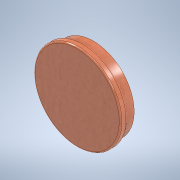
# Autodesk Inventor part: Mocowanie spadochronu
Saved by Autodesk Inventor 2020 (Build 240168000, 168)
## iProperties
Created: 2021-10-14
Part Number: Mocowanie spadochronu
Material: Ogólny
Document SubType Name: Modeling
Designer: Komputer
Density: 1 g/cm^3
Appearance: Orzech — naturalny — polerowany
Author: Komputer
Autodesk Inventor part; units mm, degrees
ref_plane "YZ Plane" through (0, 0, 0) normal (1, 0, 0) x (0, 1, 0)
ref_plane "XZ Plane" through (0, 0, 0) normal (0, 1, 0) x (-1, 0, 0)
ref_plane "XY Plane" through (0, 0, 0) normal (0, 0, 1) x (1, 0, 0)
sketch "Szkic1" plane through (0, 0, 0) normal (0, 0, 1) x (1, 0, 0)
  circle A0 centre (0, 0) radius 32
  dimension "d0" = 64
  constraints: 1 centre point, 1 coincident
  measures "d0" diameter of A0
extrude "Wyciągnięcie proste1" add sketch "Szkic1" along normal blind 5
sketch "Szkic2" plane through (0, 0, 0) normal (0, 0, -1) x (-1, 0, 0)
  circle A0 centre (0, 0) radius 5
  dimension "d3" = 10
  constraints: 1 centre point, 1 coincident
  measures "d3" diameter of A0
extrude "Wyciągnięcie proste2" add sketch "Szkic2" along normal blind 14
fillet "Zaokrąglenie1" radius 1 3 edges at (-32, 0, 0) (-32, 0, 5) (5, 0, -14)
sketch "Szkic3" plane through (0, 0, 0) normal (0, 0, -1) x (-1, 0, 0)
  circle A0 centre (0, 0) radius 27.5
  circle A1 centre (0, 0) radius 4 projected
  circle A2 centre (0, 0) radius 30
  line L0 (0, 26) -> (0.5, 26)
  line L1 (0, 26) -> (-0.5, 26)
  line L2 (-0.5, 26) -> (-1.3243, 27.4277)
  line L3 (-1.3243, 27.4277) -> (-1.347, 27.467)
  line L4 (0.5, 26) -> (1.347, 27.467)
  line L5 (-3.6185, 25.747) -> (-3.1234, 25.8166)
  line L6 (-3.6185, 25.747) -> (-4.1136, 25.6774)
  line L7 (-4.1136, 25.6774) -> (-5.1286, 26.9765)
  line L8 (-5.1286, 26.9765) -> (-5.1565, 27.0122)
  line L9 (-3.1234, 25.8166) -> (-2.4888, 27.3871)
  line L10 (-7.1666, 24.9928) -> (-6.6859, 25.1306)
  line L11 (-7.1666, 24.9928) -> (-7.6472, 24.855)
  line L12 (-7.6472, 24.855) -> (-8.8331, 26.0002)
  line L13 (-8.8331, 26.0002) -> (-8.8657, 26.0317)
  line L14 (-6.6859, 25.1306) -> (-6.2761, 26.7742)
  line L15 (-10.5752, 23.7522) -> (-10.1184, 23.9556)
  line L16 (-10.5752, 23.7522) -> (-11.0319, 23.5488)
  line L17 (-11.0319, 23.5488) -> (-12.3657, 24.5178)
  line L18 (-12.3657, 24.5178) -> (-12.4023, 24.5445)
  line L19 (-10.1184, 23.9556) -> (-9.9413, 25.6402)
  line L20 (-13.7779, 22.0493) -> (-13.3539, 22.3142)
  line L21 (-13.7779, 22.0493) -> (-14.2019, 21.7843)
  line L22 (-14.2019, 21.7843) -> (-15.6576, 22.5583)
  line L23 (-15.6576, 22.5583) -> (-15.6976, 22.5795)
  line L24 (-13.3539, 22.3142) -> (-13.413, 24.0071)
  line L25 (-16.7125, 19.9172) -> (-16.3295, 20.2385)
  line L26 (-16.7125, 19.9172) -> (-17.0955, 19.5958)
  line L27 (-17.0955, 19.5958) -> (-18.6447, 20.1596)
  line L28 (-18.6447, 20.1596) -> (-18.6873, 20.1751)
  line L29 (-16.3295, 20.2385) -> (-16.6236, 21.9068)
  line L30 (-19.3218, 17.3974) -> (-18.9872, 17.769)
  line L31 (-19.3218, 17.3974) -> (-19.6563, 17.0258)
  line L32 (-19.6563, 17.0258) -> (-21.2689, 17.3686)
  line L33 (-21.2689, 17.3686) -> (-21.3133, 17.378)
  line L34 (-18.9872, 17.769) -> (-19.5107, 19.38)
  line L35 (-21.555, 14.539) -> (-21.2754, 14.9535)
  line L36 (-21.555, 14.539) -> (-21.8346, 14.1245)
  line L37 (-21.8346, 14.1245) -> (-23.4792, 14.2395)
  line L38 (-23.4792, 14.2395) -> (-23.5244, 14.2427)
  line L39 (-21.2754, 14.9535) -> (-22.018, 16.476)
  line L40 (-23.3686, 11.3976) -> (-23.1495, 11.847)
  line L41 (-23.3686, 11.3976) -> (-23.5878, 10.9483)
  line L42 (-23.5878, 10.9483) -> (-25.2324, 10.8333)
  line L43 (-25.2324, 10.8333) -> (-25.2776, 10.8301)
  line L44 (-23.1495, 11.847) -> (-24.0967, 13.2514)
  line L45 (-24.7275, 8.0344) -> (-24.573, 8.51)
  line L46 (-24.7275, 8.0344) -> (-24.882, 7.5589)
  line L47 (-24.882, 7.5589) -> (-26.4946, 7.2161)
  line L48 (-26.4946, 7.2161) -> (-26.5389, 7.2067)
  line L49 (-24.573, 8.51) -> (-25.7064, 9.7688)
  line L50 (-25.605, 4.5149) -> (-25.5182, 5.0073)
  line L51 (-25.605, 4.5149) -> (-25.6918, 4.0224)
  line L52 (-25.6918, 4.0224) -> (-27.241, 3.4586)
  line L53 (-27.241, 3.4586) -> (-27.2836, 3.4431)
  line L54 (-25.5182, 5.0073) -> (-26.8158, 6.0961)
  line L55 (-25.9842, 0.9074) -> (-25.9667, 1.4071)
  line L56 (-25.9842, 0.9074) -> (-26.0016, 0.4077)
  line L57 (-26.0016, 0.4077) -> (-27.4573, -0.3663)
  line L58 (-27.4573, -0.3663) -> (-27.4973, -0.3876)
  line L59 (-25.9667, 1.4071) -> (-27.4033, 2.3047)
  line L60 (-25.8576, -2.7177) -> (-25.9098, -2.2205)
  line L61 (-25.8576, -2.7177) -> (-25.8053, -3.215)
  line L62 (-25.8053, -3.215) -> (-27.1391, -4.184)
  line L63 (-27.1391, -4.184) -> (-27.1757, -4.2107)
  line L64 (-25.9098, -2.2205) -> (-27.4573, -1.5315)
  line L65 (-25.2277, -6.29) -> (-25.3486, -5.8048)
  line L66 (-25.2277, -6.29) -> (-25.1067, -6.7751)
  line L67 (-25.1067, -6.7751) -> (-26.2926, -7.9203)
  line L68 (-26.2926, -7.9203) -> (-26.3252, -7.9518)
  line L69 (-25.3486, -5.8048) -> (-26.977, -5.3379)
  line L70 (-24.1068, -9.7398) -> (-24.2941, -9.2762)
  line L71 (-24.1068, -9.7398) -> (-23.9195, -10.2034)
  line L72 (-23.9195, -10.2034) -> (-24.9345, -11.5025)
  line L73 (-24.9345, -11.5025) -> (-24.9624, -11.5382)
  line L74 (-24.2941, -9.2762) -> (-25.9715, -9.0404)
  line L75 (-22.5167, -13) -> (-22.7667, -12.567)
  line L76 (-22.5167, -13) -> (-22.2667, -13.433)
  line L77 (-22.2667, -13.433) -> (-23.091, -14.8608)
  line L78 (-23.091, -14.8608) -> (-23.1136, -14.9)
  line L79 (-22.7667, -12.567) -> (-24.4606, -12.567)
  line L80 (-20.4883, -16.0072) -> (-20.7961, -15.6132)
  line L81 (-20.4883, -16.0072) -> (-20.1804, -16.4012)
  line L82 (-20.1804, -16.4012) -> (-20.798, -17.9298)
  line L83 (-20.798, -17.9298) -> (-20.815, -17.9718)
  line L84 (-20.7961, -15.6132) -> (-22.4736, -15.8489)
  line L85 (-18.0611, -18.7028) -> (-18.4208, -18.3555)
  line L86 (-18.0611, -18.7028) -> (-17.7014, -19.0502)
  line L87 (-17.7014, -19.0502) -> (-18.1003, -20.6498)
  line L88 (-18.1003, -20.6498) -> (-18.1112, -20.6938)
  line L89 (-18.4208, -18.3555) -> (-20.0491, -18.8224)
  line L90 (-15.2824, -21.0344) -> (-15.6869, -20.7405)
  line L91 (-15.2824, -21.0344) -> (-14.8779, -21.3283)
  line L92 (-14.8779, -21.3283) -> (-15.0502, -22.9679)
  line L93 (-15.0502, -22.9679) -> (-15.055, -23.013)
  line L94 (-15.6869, -20.7405) -> (-17.2344, -21.4295)
  line L95 (-12.2063, -22.9566) -> (-12.6477, -22.7219)
  line L96 (-12.2063, -22.9566) -> (-11.7648, -23.1914)
  line L97 (-11.7648, -23.1914) -> (-11.7073, -24.839)
  line L98 (-11.7073, -24.839) -> (-11.7057, -24.8843)
  line L99 (-12.6477, -22.7219) -> (-14.0843, -23.6196)
  line L100 (-8.8925, -24.432) -> (-9.3624, -24.261)
  line L101 (-8.8925, -24.432) -> (-8.4227, -24.603)
  line L102 (-8.4227, -24.603) -> (-8.1364, -26.2266)
  line L103 (-8.1364, -26.2266) -> (-8.1285, -26.2712)
  line L104 (-9.3624, -24.261) -> (-10.66, -25.3498)
  line L105 (-5.4057, -25.4318) -> (-5.8948, -25.3279)
  line L106 (-5.4057, -25.4318) -> (-4.9166, -25.5358)
  line L107 (-4.9166, -25.5358) -> (-4.4072, -27.1037)
  line L108 (-4.4072, -27.1037) -> (-4.3932, -27.1468)
  line L109 (-5.8948, -25.3279) -> (-7.0282, -26.5867)
  line L110 (-1.8137, -25.9367) -> (-2.3125, -25.9018)
  line L111 (-1.8137, -25.9367) -> (-1.3149, -25.9715)
  line L112 (-1.3149, -25.9715) -> (-0.5922, -27.4533)
  line L113 (-0.5922, -27.4533) -> (-0.5723, -27.494)
  line L114 (-2.3125, -25.9018) -> (-3.2597, -27.3061)
  line L115 (1.8137, -25.9367) -> (1.3149, -25.9715)
  line L116 (1.8137, -25.9367) -> (2.3125, -25.9018)
  line L117 (2.3125, -25.9018) -> (3.2343, -27.2686)
  line L118 (3.2343, -27.2686) -> (3.2597, -27.3061)
  line L119 (1.3149, -25.9715) -> (0.5723, -27.494)
  line L120 (5.4057, -25.4318) -> (4.9166, -25.5358)
  line L121 (5.4057, -25.4318) -> (5.8948, -25.3279)
  line L122 (5.8948, -25.3279) -> (6.9979, -26.553)
  line L123 (6.9979, -26.553) -> (7.0282, -26.5867)
  line L124 (4.9166, -25.5358) -> (4.3932, -27.1468)
  line L125 (8.8925, -24.432) -> (8.4227, -24.603)
  line L126 (8.8925, -24.432) -> (9.3624, -24.261)
  line L127 (9.3624, -24.261) -> (10.6253, -25.3207)
  line L128 (10.6253, -25.3207) -> (10.66, -25.3498)
  line L129 (8.4227, -24.603) -> (8.1285, -26.2712)
  line L130 (12.2063, -22.9566) -> (11.7648, -23.1914)
  line L131 (12.2063, -22.9566) -> (12.6477, -22.7219)
  line L132 (12.6477, -22.7219) -> (14.0458, -23.5955)
  line L133 (14.0458, -23.5955) -> (14.0843, -23.6196)
  line L134 (11.7648, -23.1914) -> (11.7057, -24.8843)
  line L135 (15.2824, -21.0344) -> (14.8779, -21.3283)
  line L136 (15.2824, -21.0344) -> (15.6869, -20.7405)
  line L137 (15.6869, -20.7405) -> (17.193, -21.4111)
  line L138 (17.193, -21.4111) -> (17.2344, -21.4295)
  line L139 (14.8779, -21.3283) -> (15.055, -23.013)
  line L140 (18.0611, -18.7028) -> (17.7014, -19.0502)
  line L141 (18.0611, -18.7028) -> (18.4208, -18.3555)
  line L142 (18.4208, -18.3555) -> (20.0055, -18.8099)
  line L143 (20.0055, -18.8099) -> (20.0491, -18.8224)
  line L144 (17.7014, -19.0502) -> (18.1112, -20.6938)
  line L145 (20.4883, -16.0072) -> (20.1804, -16.4012)
  line L146 (20.4883, -16.0072) -> (20.7961, -15.6132)
  line L147 (20.7961, -15.6132) -> (22.4287, -15.8426)
  line L148 (22.4287, -15.8426) -> (22.4736, -15.8489)
  line L149 (20.1804, -16.4012) -> (20.815, -17.9718)
  line L150 (22.5167, -13) -> (22.2667, -13.433)
  line L151 (22.5167, -13) -> (22.7667, -12.567)
  line L152 (22.7667, -12.567) -> (24.4153, -12.567)
  line L153 (24.4153, -12.567) -> (24.4606, -12.567)
  line L154 (22.2667, -13.433) -> (23.1136, -14.9)
  line L155 (24.1068, -9.7398) -> (23.9195, -10.2034)
  line L156 (24.1068, -9.7398) -> (24.2941, -9.2762)
  line L157 (24.2941, -9.2762) -> (25.9267, -9.0467)
  line L158 (25.9267, -9.0467) -> (25.9715, -9.0404)
  line L159 (23.9195, -10.2034) -> (24.9624, -11.5382)
  line L160 (25.2277, -6.29) -> (25.1067, -6.7751)
  line L161 (25.2277, -6.29) -> (25.3486, -5.8048)
  line L162 (25.3486, -5.8048) -> (26.9334, -5.3504)
  line L163 (26.9334, -5.3504) -> (26.977, -5.3379)
  line L164 (25.1067, -6.7751) -> (26.3252, -7.9518)
  line L165 (25.8576, -2.7177) -> (25.8053, -3.215)
  line L166 (25.8576, -2.7177) -> (25.9098, -2.2205)
  line L167 (25.9098, -2.2205) -> (27.4159, -1.5499)
  line L168 (27.4159, -1.5499) -> (27.4573, -1.5315)
  line L169 (25.8053, -3.215) -> (27.1757, -4.2107)
  line L170 (25.9842, 0.9074) -> (26.0016, 0.4077)
  line L171 (25.9842, 0.9074) -> (25.9667, 1.4071)
  line L172 (25.9667, 1.4071) -> (27.3648, 2.2807)
  line L173 (27.3648, 2.2807) -> (27.4033, 2.3047)
  line L174 (26.0016, 0.4077) -> (27.4973, -0.3876)
  line L175 (25.605, 4.5149) -> (25.6918, 4.0224)
  line L176 (25.605, 4.5149) -> (25.5182, 5.0073)
  line L177 (25.5182, 5.0073) -> (26.7811, 6.067)
  line L178 (26.7811, 6.067) -> (26.8158, 6.0961)
  line L179 (25.6918, 4.0224) -> (27.2836, 3.4431)
  line L180 (24.7275, 8.0344) -> (24.882, 7.5589)
  line L181 (24.7275, 8.0344) -> (24.573, 8.51)
  line L182 (24.573, 8.51) -> (25.6761, 9.7351)
  line L183 (25.6761, 9.7351) -> (25.7064, 9.7688)
  line L184 (24.882, 7.5589) -> (26.5389, 7.2067)
  line L185 (23.3686, 11.3976) -> (23.5878, 10.9483)
  line L186 (23.3686, 11.3976) -> (23.1495, 11.847)
  line L187 (23.1495, 11.847) -> (24.0714, 13.2138)
  line L188 (24.0714, 13.2138) -> (24.0967, 13.2514)
  line L189 (23.5878, 10.9483) -> (25.2776, 10.8301)
  line L190 (21.555, 14.539) -> (21.8346, 14.1245)
  line L191 (21.555, 14.539) -> (21.2754, 14.9535)
  line L192 (21.2754, 14.9535) -> (21.9981, 16.4353)
  line L193 (21.9981, 16.4353) -> (22.018, 16.476)
  line L194 (21.8346, 14.1245) -> (23.5244, 14.2427)
  line L195 (19.3218, 17.3974) -> (19.6563, 17.0258)
  line L196 (19.3218, 17.3974) -> (18.9872, 17.769)
  line L197 (18.9872, 17.769) -> (19.4967, 19.3369)
  line L198 (19.4967, 19.3369) -> (19.5107, 19.38)
  line L199 (19.6563, 17.0258) -> (21.3133, 17.378)
  line L200 (16.7125, 19.9172) -> (17.0955, 19.5958)
  line L201 (16.7125, 19.9172) -> (16.3295, 20.2385)
  line L202 (16.3295, 20.2385) -> (16.6157, 21.8621)
  line L203 (16.6157, 21.8621) -> (16.6236, 21.9068)
  line L204 (17.0955, 19.5958) -> (18.6873, 20.1751)
  line L205 (13.7779, 22.0493) -> (14.2019, 21.7843)
  line L206 (13.7779, 22.0493) -> (13.3539, 22.3142)
  line L207 (13.3539, 22.3142) -> (13.4114, 23.9618)
  line L208 (13.4114, 23.9618) -> (13.413, 24.0071)
  line L209 (14.2019, 21.7843) -> (15.6976, 22.5795)
  line L210 (10.5752, 23.7522) -> (11.0319, 23.5488)
  line L211 (10.5752, 23.7522) -> (10.1184, 23.9556)
  line L212 (10.1184, 23.9556) -> (9.9461, 25.5951)
  line L213 (9.9461, 25.5951) -> (9.9413, 25.6402)
  line L214 (11.0319, 23.5488) -> (12.4023, 24.5445)
  line L215 (7.1666, 24.9928) -> (7.6472, 24.855)
  line L216 (7.1666, 24.9928) -> (6.6859, 25.1306)
  line L217 (6.6859, 25.1306) -> (6.2871, 26.7303)
  line L218 (6.2871, 26.7303) -> (6.2761, 26.7742)
  line L219 (7.6472, 24.855) -> (8.8657, 26.0317)
  line L220 (3.6185, 25.747) -> (4.1136, 25.6774)
  line L221 (3.6185, 25.747) -> (3.1234, 25.8166)
  line L222 (3.1234, 25.8166) -> (2.5058, 27.3451)
  line L223 (2.5058, 27.3451) -> (2.4888, 27.3871)
  line L224 (4.1136, 25.6774) -> (5.1565, 27.0122)
  point P0 (27.4973, -0.3876)
  dimension "d7" = 55
  dimension "d8" = 60
  dimension "d16" = 0.5
  dimension "d17" = 0.5
  dimension "d18" = 120
  dimension "d22" = 360
  constraints: 450 end point, 45 point on line, 2 coincident, 1 centre point, 1 horizontal, 499 other
  measures "d8" diameter of A2
  measures "d16" distance of L0.start L0.end
  measures "d17" distance of L0.start L1.end
  measures "d18" angle of L1 L2
extrude "Wyciągnięcie proste3" add sketch "Szkic3" along normal blind 7 contours A0 L174 L170 L171 L172 L173 | L179 L175 L176 L177 L178 A0 | A0 L169 L165 L166 L167 L168 | L184 L180 L181 L182 L183 A0 | A0 L164 L160 L161 L162 L163 | L189 L185 L186 L187 L188 A0 | A0 L159 L155 L156 L157 L158 | L194 L190 L191 L192 L193 A0 | A0 L154 L150 L151 L152 L153 | L199 L195 L196 L197 L198 A0 | A0 L149 L145 L146 L147 L148 | L204 L200 L201 L202 L203 A0 | A0 L144 L140 L141 L142 L143 | L209 L205 L206 L207 L208 A0 | A0 L139 L135 L136 L137 L138 | L214 L210 L211 L212 L213 A0 | A0 L134 L130 L131 L132 L133 | L219 L215 L216 L217 L218 A0 | A0 L129 L125 L126 L127 L128 | L224 L220 L221 L222 L223 A0 | A0 L124 L120 L121 L122 L123 | L4 L0 L1 L2 L3 A0 | A0 L119 L115 L116 L117 L118 | L9 L5 L6 L7 L8 A0 | A0 L114 L110 L111 L112 L113 | L14 L10 L11 L12 L13 A0 | A0 L109 L105 L106 L107 L108 | L19 L15 L16 L17 L18 A0 | A0 L104 L100 L101 L102 L103 | L24 L20 L21 L22 L23 A0 | A0 L99 L95 L96 L97 L98 | L29 L25 L26 L27 L28 A0 | A0 L94 L90 L91 L92 L93 | L34 L30 L31 L32 L33 A0 | A0 L89 L85 L86 L87 L88 | L39 L35 L36 L37 L38 A0 | A0 L84 L80 L81 L82 L83 | L44 L40 L41 L42 L43 A0 | A0 L79 L75 L76 L77 L78 | L49 L45 L46 L47 L48 A0 | A0 L74 L70 L71 L72 L73 | L54 L50 L51 L52 L53 A0 | A0 L69 L65 L66 L67 L68 | L59 L55 L56 L57 L58 A0 | A0 L64 L60 L61 L62 L63 | A2
sketch "Szkic4" plane through (0, 0, -14) normal (0, 0, -1) x (-1, 0, 0)
  point P0 (0, 0)
